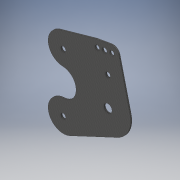
# Autodesk Inventor part: Shooter Side Plate
Saved by Autodesk Inventor 2019.4 (Build 234330000, 330)
## iProperties
Created: 2020-01-16
Part Number: Shooter Side Plate
Material: CFRP
Document SubType Name: Modeling
Designer: admin
Density: 1.43 g/cm^3
Appearance: Carbon Fiber
Mass: 608.192 g
Surface Area: 1789.71 cm^2
Volume: 425.309 cm^3
Author: admin
Autodesk Inventor part; units mm, degrees
ref_plane "YZ Plane" through (0, 0, 0) normal (1, 0, 0) x (0, 1, 0)
ref_plane "XZ Plane" through (0, 0, 0) normal (0, 1, 0) x (-1, 0, 0)
ref_plane "XY Plane" through (0, 0, 0) normal (0, 0, 1) x (1, 0, 0)
sketch "Sketch1" plane through (0, 0, 0) normal (0, 0, 1) x (1, 0, 0)
  arc A0 (86.3791, 21.0203) -> (37.691, -80.5146) centre (0, 0) ccw construction
  circle A1 centre (0, 114.3) radius 50.8 construction
  circle A2 centre (-176.0001, 114.3) radius 50.8 construction
  circle A3 centre (-176.0001, -114.3) radius 50.8 construction
  line L0 (-176.0001, 114.3) -> (-176.0001, -114.3) construction
  line L1 (-176.0001, 0) -> (0, 0) construction
  circle A4 centre (-176.0001, -114.3) radius 9.5
  circle A5 centre (-176.0001, 114.3) radius 9.5
  circle A6 centre (0, 114.3) radius 9.5
  line L2 (0, 0) -> (0, 114.3) construction
  circle A7 centre (-42.062, 186.0077) radius 9
  circle A8 centre (15.5014, 195.9756) radius 9
  line L3 (0, 114.3) -> (15.5014, 195.9756) construction
  line L4 (0, 114.3) -> (-42.062, 186.0077) construction
  arc A9 (10.8092, 223.0724) -> (42.2216, 202.478) centre (15.5014, 195.9756) ccw construction
  arc A10 (-49.555, 212.4672) -> (-46.7542, 213.1044) centre (-42.062, 186.0077) ccw construction
  line L5 (0, 0) -> (-490.9821, 0) construction
  line L6 (42.2216, 202.478) -> (86.3791, 21.0203)
  line L7 (-46.7542, 213.1044) -> (10.8092, 223.0724)
  arc A11 (-192.3484, 172.0298) -> (-178.0985, 54.3367) centre (-176.0001, 114.3) ccw
  arc A12 (-178.0985, -54.3367) -> (-150.5618, -168.6406) centre (-176.0001, -114.3) ccw
  line L8 (-192.3484, 172.0298) -> (-49.555, 212.4672)
  line L9 (-150.5618, -168.6406) -> (37.691, -80.5146)
  arc A13 (-178.0985, -54.3367) -> (-178.0985, 54.3367) centre (-180, 0) ccw
  arc A14 (37.691, -80.5146) -> (86.3791, 21.0203) centre (0, 0) ccw
  arc A15 (-178.0985, 54.3367) -> (-192.3484, 172.0298) centre (-176.0001, 114.3) ccw construction
  arc A16 (-150.5618, -168.6406) -> (-178.0985, -54.3367) centre (-176.0001, -114.3) ccw construction
  circle A17 centre (0, 0) radius 16
  line L10 (-176.0001, -114.3) -> (0, 114.3) construction
  line L11 (-176.0001, 114.3) -> (-118.4041, 192.9699) construction
  circle A18 centre (-13.2803, 190.9917) radius 22.86 construction
  circle A19 centre (-42.062, 186.0077) radius 6.35 construction
  circle A20 centre (15.5014, 195.9756) radius 6.35 construction
  line L12 (-42.062, 186.0077) -> (15.5014, 195.9756) construction
  arc A21 (-46.7542, 213.1044) -> (-49.555, 212.4672) centre (-42.062, 186.0077) ccw
  arc A22 (42.2216, 202.478) -> (10.8092, 223.0724) centre (15.5014, 195.9756) ccw
  circle A23 centre (-13.2803, 190.9917) radius 9.5
  line L13 (0, 114.3) -> (-13.2803, 190.9917) construction
  line L14 (-13.2803, 190.9917) -> (-176.0001, 114.3) construction
  dimension "d37" = 177.8
  dimension "d38" = 101.6
  dimension "d39" = 101.6
  dimension "d40" = 101.6
  dimension "d41" = 19
  dimension "d42" = 19
  dimension "d43" = 19
  dimension "d44" = 114.3
  dimension "d46" = 228.6
  dimension "d47" = 18
  dimension "d48" = 18
  dimension "d50" = 55
  dimension "d52" = 55
  dimension "d54" = 0
  dimension "d55" = 176.0001
  dimension "d58" = 120
  dimension "d59" = 120
  dimension "d60" = 180
  dimension "d61" = 32
  dimension "d64" = 288.503
  dimension "d67" = 97.5
  dimension "d77" = 45.72
  dimension "d78" = 12.7
  dimension "d79" = 12.7
  dimension "d80" = 19
  dimension "d81" = 77.833
  dimension "d82" = 179.887
  constraints: 30 end point, 24 centre point, 22 point on circle, 11 coincident, 11 tangent, 2 midpoint, 2 perpendicular, 2 point on line, 1 equal length, 1 horizontal
  measures "d37" diameter of A0
  measures "d38" diameter of A1
  measures "d39" diameter of A2
  measures "d40" diameter of A3
  measures "d41" diameter of A4
  measures "d42" diameter of A5
  measures "d43" diameter of A6
  measures "d44" distance of L1.end L2.end
  measures "d46" distance of L0.start L0.end
  measures "d47" diameter of A7
  measures "d48" diameter of A8
  measures "d50" diameter of A9
  measures "d52" diameter of A10
  measures "d54" distance between parallel lines of L1 L5
  measures "d55" distance from line of point (0, 0) L0
  measures "d58" diameter of A11
  measures "d59" diameter of A12
  measures "d60" distance of point (0, 0) A13.centre
  measures "d61" diameter of A17
  measures "d64" distance of L10.start L2.end
  measures "d67" distance of L11.start L11.end
  measures "d77" diameter of A18
  measures "d78" diameter of A19
  measures "d79" diameter of A20
  measures "d80" diameter of A23
  measures "d81" distance of L2.end L13.end
  measures "d82" distance of L13.end L11.start
extrude "Extrusion1" add sketch "Sketch1" along normal blind 5
sketch "Sketch4" plane through (0, 0, 5) normal (0, 0, 1) x (1, 0, 0)
  circle A0 centre (0, 0) radius 16 projected
  circle A1 centre (-13.2803, 190.9917) radius 9.5 projected
  circle A2 centre (0, 114.3) radius 9.5 projected
  circle A3 centre (-176.0001, 114.3) radius 9.5 projected
  circle A4 centre (-176.0001, -114.3) radius 9.5 projected
  circle A5 centre (15.5014, 195.9756) radius 9 projected
  circle A6 centre (-42.062, 186.0077) radius 9 projected
  line L0 (86.3791, 21.0203) -> (42.2216, 202.478) projected
  arc A7 (42.2216, 202.478) -> (10.8092, 223.0724) centre (15.5014, 195.9756) ccw projected
  line L1 (10.8092, 223.0724) -> (-46.7542, 213.1044) projected
  arc A8 (-46.7542, 213.1044) -> (-49.555, 212.4672) centre (-42.062, 186.0077) ccw projected
  line L2 (-49.555, 212.4672) -> (-192.3484, 172.0298) projected
  arc A9 (-192.3484, 172.0298) -> (-178.0985, 54.3367) centre (-176.0001, 114.3) ccw projected
  arc A10 (-178.0985, -54.3367) -> (-178.0985, 54.3367) centre (-180, 0) ccw projected
  arc A11 (-178.0985, -54.3367) -> (-150.5618, -168.6406) centre (-176.0001, -114.3) ccw projected
  line L3 (-150.5618, -168.6406) -> (37.691, -80.5146) projected
  arc A12 (37.691, -80.5146) -> (86.3791, 21.0203) centre (0, 0) ccw projected
  line L4 (-186.899, 152.7865) -> (-44.1055, 193.2239)
  arc A13 (-43.3416, 193.3977) -> (-44.1055, 193.2239) centre (-42.062, 186.0077) ccw
  line L5 (-43.3416, 193.3977) -> (14.2217, 203.3656)
  arc A14 (22.7887, 197.749) -> (14.2217, 203.3656) centre (15.5014, 195.9756) ccw
  line L6 (22.7887, 197.749) -> (66.9463, 16.2913)
  arc A15 (29.2115, -62.4011) -> (66.9463, 16.2913) centre (0, 0) ccw
  line L7 (29.2115, -62.4011) -> (-159.0413, -150.527)
  arc A16 (-177.399, -74.3245) -> (-159.0413, -150.527) centre (-176.0001, -114.3) ccw
  arc A17 (-177.399, -74.3245) -> (-177.399, 74.3245) centre (-180, 0) ccw
  arc A18 (-186.899, 152.7865) -> (-177.399, 74.3245) centre (-176.0001, 114.3) ccw
  line L8 (-65.3945, 187.1951) -> (-57.3771, 158.8839)
  line L9 (-57.3771, 158.8839) -> (27.2358, 179.4744)
  circle A19 centre (0, 114.3) radius 24.5
  circle A20 centre (-176.0001, 114.3) radius 29.5
  circle A21 centre (0, 0) radius 36
  circle A22 centre (-176.0001, -114.3) radius 29.5
  line L10 (-196.7466, -93.3278) -> (-203.7984, -85.538)
  line L11 (-189.0882, -76.5018) -> (-181.1639, -85.2555)
  line L12 (-205.5001, -114.3) -> (-215.0539, -122.9486)
  line L13 (-197.87, -134.0979) -> (-205.6542, -141.1446)
  line L14 (-176.0001, -143.8) -> (-167.3514, -153.3538)
  line L15 (-156.2022, -136.1699) -> (-147.9188, -145.3203)
  line L16 (-137.3202, -60.9042) -> (-78.037, -112.6069)
  line L17 (-113.8583, -34.0025) -> (-42.062, -95.766)
  dimension "d83" = 20
  dimension "d84" = 15
  dimension "d85" = 20
  dimension "d86" = 20
  dimension "d87" = 20
  constraints: 28 end point, 25 point on circle, 10 centre point, 5 point on line, 4 parallel, 3 perpendicular, 2 line through centre, 9 other
  measures "d83" distance between parallel lines of L2 L4
  measures "d84" radial gap between concentric circles of A2 A19
  measures "d85" radial gap between concentric circles of A3 A20
  measures "d86" radial gap between concentric circles of A0 A21
  measures "d87" radial gap between concentric circles of A4 A22
body "Solid1"
